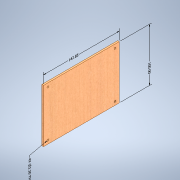
# Autodesk Inventor part: VP-01
Saved by Autodesk Inventor 2022 (Build 260153000, 153)
## iProperties
Company: El Camino College
Created: 2023-03-29
Part Number: VP-01
Material: Wood (Cherry)
Document SubType Name: Modeling
Designer: Edgar Tejada
Density: 0.63 g/cm^3
Appearance: Cherry - Natural Low Gloss
Project: Ergonomic Fight Stick
Mass: 28.5051 g
Surface Area: 301.753 cm^2
Volume: 45.2463 cm^3
Author: Edgar Tejada
Title: Vertical Plate
Subject: Ergonomic Fight Stick
Autodesk Inventor part; units mm, degrees
ref_plane "YZ Plane" through (0, 0, 0) normal (1, 0, 0) x (0, 1, 0)
ref_plane "XZ Plane" through (0, 0, 0) normal (0, 1, 0) x (-1, 0, 0)
ref_plane "XY Plane" through (0, 0, 0) normal (0, 0, 1) x (1, 0, 0)
sketch "Sketch1" plane through (0, 0, 0) normal (1, 0, 0) x (0, 1, 0)
  line L0 (50, 71.425) -> (-50, 71.425)
  line L1 (-50, 71.425) -> (-50, -71.425)
  line L2 (-50, -71.425) -> (50, -71.425)
  line L3 (50, -71.425) -> (50, 71.425)
  line L4 (50, 71.425) -> (-50, -71.425) construction
  line L5 (-50, 71.425) -> (50, -71.425) construction
  point P0 (0, 0)
  constraints: 12 end point, 2 midpoint, 2 parallel, 1 horizontal, 1 horizontal alignment, 1 perpendicular, 1 vertical alignment
extrude "Side_Base" add sketch "Sketch1" along normal blind 3.175
sketch "Sketch2" plane through (3.175, 0, 0) normal (1, 0, 0) x (0, 0, -1)
  circle A0 centre (-63.275, 43.4) radius 1.65
  circle A1 centre (63.205, 43.4) radius 1.65
  circle A2 centre (63.205, -43.4) radius 1.65
  circle A3 centre (-63.275, -43.4) radius 1.65
  line L0 (71.425, 50) -> (-71.425, 50) projected
  line L1 (-71.425, 50) -> (-71.425, -50) projected
  line L2 (71.425, -50) -> (71.425, 50) projected
  line L3 (-71.425, -50) -> (71.425, -50) projected
  point P0 (0, 0)
  dimension "d5" = 6.6
  dimension "d6" = 8.15
  dimension "d8" = 6.6
  dimension "d19" = 126.48
  dimension "d20" = 8.22
  constraints: 4 centre point, 3 equal radius, 2 horizontal alignment, 2 vertical alignment, 1 other
  measures "d5" distance from line of L0 A0.centre
  measures "d6" distance from line of L1 A0.centre
  measures "d8" distance from line of L3 A2.centre
  measures "d19" distance of A1.centre A0.centre
  measures "d20" distance from line of L2 A1.centre
extrude "Joint_Holes" cut sketch "Sketch2" along normal through all both and the other way through all contours A0 | A1 | A2 | A3
equation "\"d8\" = d5"
body "Solid1"
